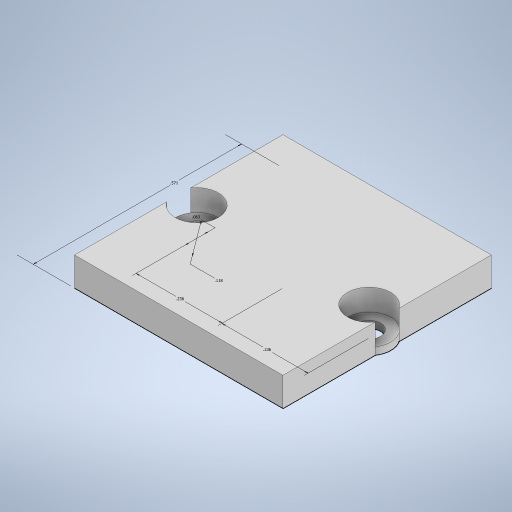
# Autodesk Inventor part: temp apd reinforcement
Saved by Autodesk Inventor 2024 (Build 280153000, 153)
## iProperties
Created: 2024-11-13
Part Number: temp apd reinforcement
Material: Generic
Document SubType Name: Modeling
Designer: Williamow
Density: 1 g/cm^3
Appearance: Default
Author: Williamow
Autodesk Inventor part; units mm, degrees
ref_plane "YZ Plane" through (0, 0, 0) normal (1, 0, 0) x (0, 1, 0)
ref_plane "XZ Plane" through (0, 0, 0) normal (0, 1, 0) x (-1, 0, 0)
ref_plane "XY Plane" through (0, 0, 0) normal (0, 0, 1) x (1, 0, 0)
sketch "Sketch1" plane through (0, 0, 0) normal (0, 1, 0) x (-1, 0, 0)
  line L0 (7.25, 7.25) -> (-7.25, 7.25)
  line L1 (-7.25, 7.25) -> (-7.25, -7.25)
  line L2 (-7.25, -7.25) -> (7.25, -7.25)
  line L3 (7.25, -7.25) -> (7.25, 7.25)
  circle A0 centre (6, 0) radius 0.8
  circle A1 centre (-6, 0) radius 0.8
  circle A2 centre (6, 0) radius 1.5
  circle A3 centre (-6, 0) radius 1.5
  point P0 (0, 0)
  point P1 (7.25, 0)
  point P2 (0, -7.25)
  dimension "d0" = 14.5
  dimension "d1" = 1.6
  dimension "d3" = 3
  dimension "d4" = 6
  dimension "d5" = 6
  constraints: 8 end point, 4 centre point, 3 horizontal alignment, 2 coincident, 2 equal radius, 2 midpoint, 2 parallel, 2 perpendicular, 1 horizontal, 1 vertical alignment
  measures "d0" distance of L2.end L0.start
  measures "d1" diameter of A0
  measures "d3" diameter of A2
  measures "d4" distance of point (0, 0) A0.centre
  measures "d5" distance of point (0, 0) A1.centre
extrude "Extrusion1" add sketch "Sketch1" along normal blind 2 contours L3 A2 L2 L1 A3 L0
extrude "Extrusion2" add sketch "Sketch1" along normal blind 0.5 contours A2 L3 | L3 A2 | A3 L1 | L1 A3
body "Solid1"
